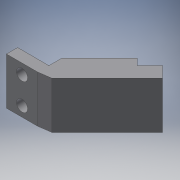
# Autodesk Inventor part: hall follower
Saved by Autodesk Inventor 2017 SP1 (Build 210196100, 196)
## iProperties
Created: 2018-02-15
Part Number: hall follower
Material: Generic
Document SubType Name: Modeling
Designer: RLanting
Density: 1 g/cm^3
Appearance: Default
Author: RLanting
Autodesk Inventor part; units mm, degrees
ref_plane "YZ Plane" through (0, 0, 0) normal (1, 0, 0) x (0, 1, 0)
ref_plane "XZ Plane" through (0, 0, 0) normal (0, 1, 0) x (-1, 0, 0)
ref_plane "XY Plane" through (0, 0, 0) normal (0, 0, 1) x (1, 0, 0)
sketch "Sketch1" plane through (0, 0, 0) normal (0, 0, 1) x (1, 0, 0)
  line L0 (0, 0) -> (-22.6274, 22.6274) construction
  circle A0 centre (0, 0) radius 32 construction
  line L1 (-31, 0) -> (-45, 0) construction
  line L2 (-45, 0) -> (-45, 19) construction
  line L3 (-45, 19) -> (-31, 19) construction
  line L4 (-31, 19) -> (-31, 0) construction
  line L5 (-31, 0) -> (0, 0) construction
  circle A1 centre (0, 0) radius 30 construction
  line L6 (-22.6274, 22.6274) -> (-0.7071, 44.5477)
  line L7 (-0.7071, 44.5477) -> (-2.1213, 45.9619)
  line L8 (-2.1213, 45.9619) -> (-24.0416, 24.0416)
  line L9 (-24.0416, 24.0416) -> (-22.6274, 22.6274)
  line L10 (-24.0416, 24.0416) -> (-22.6274, 22.6274)
  line L11 (-22.6274, 22.6274) -> (-25.4558, 19.799)
  line L12 (-25.4558, 19.799) -> (-26.8701, 21.2132)
  line L13 (-26.8701, 21.2132) -> (-24.0416, 24.0416)
  line L14 (-25.4558, 19.799) -> (-31, 19)
  line L15 (-31, 19) -> (-45, 19)
  line L16 (-45, 19) -> (-45, 24)
  line L17 (-45, 24) -> (-24.0833, 24)
  line L18 (-26.8701, 21.2132) -> (-24.0833, 24)
  line L19 (-0.7071, 44.5477) -> (0, 44.5477)
  line L20 (0, 44.5477) -> (0, 32)
  arc A2 (0, 32) -> (-22.6274, 22.6274) centre (0, 0) ccw
  point P0 (0, 38.2739)
  dimension "d0" = 19
  dimension "d1" = 31
  dimension "d2" = 14
  dimension "d4" = 60
  dimension "d5" = 2
  dimension "d6" = 2
  dimension "d8" = 4
  dimension "d9" = 35
  dimension "d10" = 45
  dimension "d13" = 5
  constraints: 42 end point, 8 equal length, 5 perpendicular, 4 point on circle, 3 centre point, 3 coincident, 3 horizontal, 1 midpoint, 1 point on line, 1 tangent, 1 vertical, 1 vertical alignment
  measures "d0" distance of L3.end L1.start
  measures "d1" distance of L1.start L5.end
  measures "d2" distance of L2.end L3.end
  measures "d4" diameter of A1
  measures "d5" radial gap between concentric circles of A1 A0
  measures "d6" distance of L6.end L7.end
  measures "d8" distance of L12.end L8.end
  measures "d9" distance between parallel lines of L7 L12
  measures "d10" angle of L5 L0
  measures "d13" distance of L2.end L16.end
extrude "Extrusion1" add sketch "Sketch1" along normal blind 21
sketch "Sketch2" plane through (-24.0833, 24, 0) normal (-0.7071068, 0.7071068, 0) x (-0.7071068, -0.7071068, 0)
  line L0 (-31.0589, 0) -> (-31.0589, 21) construction
  line L1 (-31.0589, 2) -> (-11.0589, 2)
  line L2 (-11.0589, 2) -> (-11.0589, 19)
  line L3 (-11.0589, 19) -> (-31.0589, 19)
  line L4 (-31.0589, 19) -> (-31.0589, 2)
  line L5 (-31.0589, 0) -> (0, 0) construction
  line L6 (-31.0589, 21) -> (0, 21) construction
  line L7 (-31.0589, 2) -> (-31.0589, 0)
  line L8 (0, 0) -> (0, 21) projected
  line L9 (-31.0589, 0) -> (0, 0)
  line L10 (0, 0) -> (0, 21)
  line L11 (0, 21) -> (-31.0589, 21)
  line L12 (-31.0589, 21) -> (-31.0589, 19)
  point P0 (-0.0589, 0)
  point P1 (-31.0589, 10.5)
  dimension "d14" = 17
  dimension "d15" = 20
  constraints: 18 end point, 3 collinear, 3 perpendicular, 2 midpoint, 2 parallel, 1 horizontal, 1 point on line
  measures "d14" distance of L1.end L2.end
  measures "d15" distance of L1.start L1.end
extrude "Extrusion2" add sketch "Sketch2" along normal blind 5 contours L1 L2 L3 L12 L11 L8 L9 L7
sketch "Sketch3" plane through (-16.2635, 31.8198, 2) normal (0.7071068, 0.7071068, 0) x (-0.7071068, 0.7071068, 0)
  line L0 (0, 0) -> (0, 17) construction
  line L1 (0, 0) -> (5, 0) construction
  line L2 (5, 17) -> (5, 0) construction
  line L3 (0, 17) -> (5, 17) construction
  line L4 (5, 5.5) -> (0, 5.5)
  line L5 (0, 5.5) -> (0, 11.5)
  line L6 (0, 11.5) -> (5, 11.5)
  line L7 (5, 11.5) -> (5, 5.5)
  line L8 (0, 0) -> (0, 17) projected
  point P0 (-34, -2)
  point P1 (5, 8.5)
  point P2 (0, 8.5)
  dimension "d18" = 6
  constraints: 8 end point, 4 midpoint, 2 parallel, 1 horizontal, 1 perpendicular
  measures "d18" distance between parallel lines of L6 L4
sketch "Sketch4" plane through (0, 0, 21) normal (0, 0, 1) x (1, 0, 0)
  line L0 (-24.0833, 24) -> (-45, 24) projected
  line L1 (-45, 24) -> (-45, 19) projected
  line L2 (-45, 19) -> (-31, 19) projected
  line L3 (-31, 19) -> (-25.4558, 19.799) projected
  line L4 (-25.4558, 19.799) -> (-22.6274, 22.6274) projected
  line L5 (-0.7071, 44.5477) -> (-5.6569, 49.4975) projected
  line L6 (-27.6188, 27.5355) -> (-5.6569, 49.4975) projected
  line L7 (-24.0833, 24) -> (-27.6188, 27.5355) projected
  line L8 (-11.3137, 43.8406) -> (-14.1421, 46.669)
  line L9 (-14.1421, 46.669) -> (-31, 29.8112)
  line L10 (-31, 29.8112) -> (-31, 24)
  arc A0 (0, 32) -> (-22.6274, 22.6274) centre (0, 0) ccw projected
  line L11 (0, 32) -> (0, 44.5477) projected
  line L12 (0, 44.5477) -> (-0.7071, 44.5477) projected
  dimension "d19" = 8
  dimension "d20" = 4
  constraints: 6 end point, 3 perpendicular, 2 point on line, 1 vertical alignment
  measures "d19" distance between parallel lines of L5 L8
  measures "d20" distance of L8.start L8.end
extrude "Extrusion3" add sketch "Sketch4" against normal up to surface (21 mm away) contours L0 L10 L9 L8 L6 L7
extrude "Extrusion4" cut sketch "Sketch3" against normal blind 17
sketch "Sketch5" plane through (-45, 24, 21) normal (0, 1, 0) x (1, 0, 0)
  line L0 (14, 0) -> (14, 7.5) construction
  line L1 (14, 21) -> (0, 21) construction
  line L2 (0, 21) -> (0, 0) construction
  line L3 (14, 0) -> (0, 0) construction
  line L4 (0, 21) -> (0, 0) construction
  line L5 (0, 10.5) -> (14, 10.5) construction
  line L6 (14, 0) -> (14, 21) construction
  line L7 (7, 16.5) -> (7, 4.5) construction
  circle A0 centre (7, 16.5) radius 2.5
  circle A1 centre (7, 4.5) radius 2.5
  line L8 (13.8457, 13.5) -> (14, 13.5) projected
  line L9 (14, 13.5) -> (14, 21) projected
  line L10 (14, 7.5) -> (13.8457, 7.5) projected
  line L11 (13.8457, 7.5) -> (13.8457, 13.5) projected
  point P0 (45, 21)
  point P1 (7, 10.5)
  dimension "d25" = 5
  dimension "d26" = 12
  constraints: 4 end point, 4 midpoint, 2 centre point, 2 coincident, 1 equal radius, 1 vertical
  measures "d25" diameter of A0
  measures "d26" distance of L7.start L7.end
extrude "Extrusion5" cut sketch "Sketch5" against normal through all
body "Solid1"
